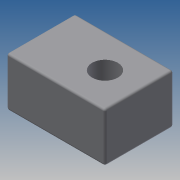
# Autodesk Inventor part: heat block
Saved by Autodesk Inventor 2013 (Build 170138000, 138)
## iProperties
Created: 2017-04-01
Part Number: heat block
Material: Generic
Document SubType Name: Modeling
Designer: employee
Density: 1 g/cm^3
Author: employee
Autodesk Inventor part; units mm, degrees
ref_plane "YZ Plane" through (0, 0, 0) normal (1, 0, 0) x (0, 1, 0)
ref_plane "XZ Plane" through (0, 0, 0) normal (0, 1, 0) x (-1, 0, 0)
ref_plane "XY Plane" through (0, 0, 0) normal (0, 0, 1) x (1, 0, 0)
sketch "Sketch1" plane through (0, 0, 0) normal (0, 0, 1) x (1, 0, 0)
  line L0 (-11.5, 8) -> (11.5, 8)
  line L1 (11.5, 8) -> (11.5, -8)
  line L2 (11.5, -8) -> (-11.5, -8)
  line L3 (-11.5, -8) -> (-11.5, 8)
  circle A0 centre (3.5, 0) radius 3
  point P0 (0, 0)
  point P1 (0, 8)
  point P2 (-11.5, 0)
  dimension "d0" = 23
  dimension "d2" = 16
  dimension "d3" = 6
  dimension "d4" = 8
  constraints: 8 end point, 2 horizontal alignment, 2 midpoint, 2 parallel, 1 centre point, 1 horizontal, 1 perpendicular, 1 vertical alignment
  measures "d0" distance of L0.start L0.end
  measures "d2" distance of L2.end L0.start
  measures "d3" diameter of A0
  measures "d4" distance from line of A0.centre L1
extrude "Extrusion1" add sketch "Sketch1" along normal blind 11.5
fillet "Fillet1" radius 0.5 12 edges at (0, 8, 11.5) (-11.5, 0, 11.5) (0, -8, 11.5) (11.5, 0, 11.5) (0, 8, 0) (-11.5, 8, 5.75) (11.5, 8, 5.75) (0, -8, 0) (11.5, -8, 5.75) (-11.5, -8, 5.75) (11.5, 0, 0) (-11.5, 0, 0)
body "Solid1"
